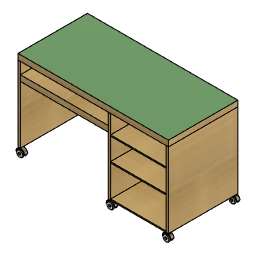
Ejercicio03jaalobuela (Autodesk Fusion 360 design; units mm, degrees)
Autodesk Fusion 360 part; units mm, degrees
box "BoxPrimitive1" add length 5 width 130 height 60 placed x (0, 0, -1) y (0, 1, 0) z (1, 0, 0) at (0, 20, 40) makes body 1
box "BoxPrimitive2" add length 70 width 60 height 2 placed x (0, 0, -1) y (-1, 0, 0) z (0, 1, 0) at (50, 0, 10) separate body makes body 2
move_body "Move1" bodies 2 to x (1, 0, 0) y (0, 1, 0) z (0, 0, 1) at (10, 20, 25)
copy_body "CopyPasteBodies1" bodies 2 makes body 3
move_body "Move2" bodies 3 to x (1, 0, 0) y (0, 1, 0) z (0, 0, 1) at (0, 128, 0)
copy_body "CopyPasteBodies2" bodies 3 makes body 4
move_body "Move3" bodies 4 to x (1, 0, 0) y (0, 1, 0) z (0, 0, 1) at (0, -50, 0)
box "BoxPrimitive3" add length 65 width 126 height 2 placed x (0, 0, -1) y (0, 1, 0) z (1, 0, 0) at (0, -161, 30) separate body makes body 5
move_body "Move4" bodies 4 to x (1, 0, 0) y (0, 1, 0) z (0, 0, 1) at (0, 0, -20)
extrude "Extrude1" cut 1 faces at (0, 98.6667, -31.6667) along direction (1, 0, 0) blind 0.2 on bodies 4 bodies 4
move_body "Move5" bodies 4 to x (1, 0, 0) y (0, 1, 0) z (0, 0, 1) at (0, 0, 20)
move_body "Move6" bodies 5 to x (1, 0, 0) y (0, 1, 0) z (0, 0, 1) at (0, 183, 5)
move_body "Move7" bodies 4 3 2 to x (1, 0, 0) y (0, 1, 0) z (0, 0, 1) at (0, 0, -75)
extrude "Extrude2" cut 3 faces at (40, 20.6667, -110) (40.0667, 98.6667, -110) (40, 148.6667, -110) along direction (0, 0, 1) blind 5 on bodies 2 3 4 bodies 2 3 4
move_body "Move8" bodies 2 3 4 to x (1, 0, 0) y (0, 1, 0) z (0, 0, 1) at (0, 0, 75)
box "BoxPrimitive4" add length 50 width 58 height 2 placed x (0, 1, 0) y (-1, 0, 0) z (0, 0, 1) at (88, 190, 0) separate body makes body 6
move_body "Move9" bodies 6 to x (1, 0, 0) y (0, 1, 0) z (0, 0, 1) at (0, -91, 0)
move_body "Move10" bodies 6 to x (1, 0, 0) y (0, 1, 0) z (0, 0, 1) at (-28, -1, -32)
move_body "Move11" bodies 6 to x (1, 0, 0) y (0, 1, 0) z (0, 0, 1) at (0, 0, -9)
extrude "Extrude3" cut 1 faces at (40.6667, 98, -40.3333) along direction (0, 1, 0) blind 2 on bodies 6 bodies 6
extrude "Extrude4" cut 1 faces at (21.3333, 116, -39) along direction (0, 0, -1) blind 1 on bodies 6 bodies 6
move_body "Move12" bodies 6 to x (1, 0, 0) y (0, 1, 0) z (0, 0, 1) at (0, 0, 11)
copy_body "CopyPasteBodies3" bodies 6 makes body 7
move_body "Move13" bodies 7 to x (1, 0, 0) y (0, 1, 0) z (0, 0, 1) at (0, 0, 28)
copy_body "CopyPasteBodies4" bodies 7 makes body 8
move_body "Move14" bodies 8 to x (1, 0, 0) y (0, 1, 0) z (0, 0, 1) at (0, 0, 20)
box "BoxPrimitive5" add length 76 width 58 height 5 placed x (0, 1, 0) y (-1, 0, 0) z (0, 0, 1) at (188, 60, 0) separate body makes body 9
move_body "Move15" bodies 9 to x (1, 0, 0) y (0, 1, 0) z (0, 0, 1) at (-128, -38, 30)
move_body "Move16" bodies 9 to x (1, 0, 0) y (0, 1, 0) z (0, 0, 1) at (0, 0, -10)
cylinder "CylinderPrimitive1" add diameter 6 height 4 placed x (0, 0, -1) y (0, 1, 0) z (1, 0, 0) at (0, 20, -33) separate body makes body 10
move_body "Move17" bodies 10 to x (1, 0, 0) y (0, 1, 0) z (0, 0, 1) at (75, 0, 0)
cylinder "CylinderPrimitive2" add diameter 2 height 4.5 placed x (0, 0, -1) y (0, 1, 0) z (1, 0, 0) at (79, 28, -25) separate body makes body 11
move_body "Move18" bodies 11 to x (1, 0, 0) y (0, 1, 0) z (0, 0, 1) at (-4.5, -8, -8)
move_body "Move19" bodies 11 to x (1, 0, 0) y (0, 1, 0) z (0, 0, 1) at (0.25, 0, 0)
box "BoxPrimitive6" add length 3 width 5 height 1 placed x (0, 1, 0) y (-1, 0, 0) z (0, 0, 1) at (131, -2, 0) separate body makes body 12
cylinder "CylinderPrimitive3" add diameter 7.5 height 4 placed x (0, 0, -1) y (0, 1, 0) z (1, 0, 0) at (0, 63, -66) separate body makes body 13
hole "Hole1" at (4, 63, -66) direction (-1, 0, 0) diameter 6 end through all bodies 13
sketch "Sketch10" plane through (4, 0, 0) normal (1, 0, 0) x (0, 1, 0)
  circle A0 centre (63, -66) radius 3
  circle A1 centre (63, -66) radius 3.75
  line L0 (58, -66) -> (70.6215, -66)
  line L1 (70.6215, -66) -> (70.6215, -70.5064)
  line L2 (70.6215, -70.5064) -> (58, -70.5064)
  line L3 (58, -70.5064) -> (58, -66)
  constraint horizontal L0
  constraint vertical L1
  constraint horizontal L2
  constraint vertical L3
move_body "Move20" bodies 13 to x (1, 0, 0) y (0, 1, 0) z (0, 0, 1) at (-2, 0, 0)
extrude "Extrude5" cut sketch "Sketch10" against normal blind 8.5 contours A0 A1 L0 | A0 L0 | A1 L0 L1 L2 L3 picked at (66.2763, -67.2056) picked at (62.6347, -68.0575) bodies 13
fillet "Fillet1" radius 0.5 1 edges at (79, 18.9152, -30.203) on bodies 10
fillet "Fillet2" radius 0.5 1 edges at (75, 21.0848, -30.203) on bodies 10
fillet "Fillet3" radius 0.2 1 edges at (79.25, 19.6384, -32.0677) on bodies 11
fillet "Fillet4" radius 0.2 1 edges at (74.75, 20.3616, -32.0677) on bodies 11
move_body "Move21" bodies 13 to x (1, 0, 0) y (0, 1, 0) z (0, 0, 1) at (76.5, -43, 30)
move_body "Move22" bodies 13 to x (1, 0, 0) y (0, 1, 0) z (0, 0, 1) at (0, 0, 3)
move_body "Move23" bodies 13 to x (1, 0, 0) y (0, 1, 0) z (0, 0, 1) at (0, 0, 4)
extrude "Extrude6" cut 1 faces at (78.5, 16.94, -27.3196) along direction (-1, 0, 0) blind 1 on bodies 13 bodies 13
move_body "Move24" bodies 13 to x (1, 0, 0) y (0, 1, 0) z (0, 0, 1) at (1, 0, -4)
fillet "Fillet5" radius 0.2 4 edges at (78.5, 20, -29.25) (77, 23.75, -33) (75.5, 20, -29.25) (77, 16.25, -33) on bodies 13
move_body "Move25" bodies 12 to x (1, 0, 0) y (0, 1, 0) z (0, 0, 1) at (-50.2, 22, -33)
move_body "Move26" bodies 12 to x (1, 0, 0) y (0, 1, 0) z (0, 0, 1) at (0, 0, 3)
move_body "Move27" bodies 12 to x (1, 0, 0) y (0, 1, 0) z (0, 0, 1) at (-2, -0.5, 1.5)
extrude "Extrude7" cut 1 faces at (73.8, 21.5, -28.1667) along direction (1, 0, 0) blind 2 on bodies 12 bodies 12
extrude "Extrude8" cut 1 faces at (76.8, 20.5, -27.5) along direction (0, 0, -1) blind 0.5 on bodies 12 bodies 12
move_body "Move28" bodies 12 to x (1, 0, 0) y (0, 1, 0) z (0, 0, 1) at (0, -0.5, -0.5)
extrude "Extrude9" add 1 faces at (77.8, 19, -28.8333) along direction (0, -1, 0) blind 0.5 on bodies 12 bodies 12
move_body "Move29" bodies 12 13 10 11 to x (1, 0, 0) y (0, 1, 0) z (0, 0, 1) at (-18, 0, -3.5)
move_body "Move30" bodies 12 to x (1, 0, 0) y (0, 1, 0) z (0, 0, 1) at (0, 0, -0.25)
move_body "Move31" bodies 12 11 13 10 to x (1, 0, 0) y (0, 1, 0) z (0, 0, 1) at (-0.8, 1.5, 2.25)
copy_body "CopyPasteBodies5" bodies 13 10 11 12 makes body 14 makes body 15 makes body 16 makes body 17
move_body "Move32" bodies 14 15 16 17 to x (1, 0, 0) y (0, 1, 0) z (0, 0, 1) at (-57, 0, 0)
copy_body "CopyPasteBodies6" bodies 13 10 11 makes body 18 makes body 19 makes body 20
move_body "Move33" bodies 18 19 20 12 to x (1, 0, 0) y (0, 1, 0) z (0, 0, 1) at (0, 78, 0)
copy_body "CopyPasteBodies7" bodies 20 18 19 12 makes body 21 makes body 22 makes body 23 makes body 24
move_body "Move34" bodies 21 22 23 24 to x (1, 0, 0) y (0, 1, 0) z (0, 0, 1) at (0, 48.5, 0)
copy_body "CopyPasteBodies8" bodies 22 21 23 18 19 20 24 12 makes body 25 makes body 26 makes body 27 makes body 28 makes body 29 makes body 30 makes body 31 makes body 32
move_body "Move35" bodies 25 26 27 28 29 30 31 32 to x (1, 0, 0) y (0, 1, 0) z (0, 0, 1) at (-60, 0, 0)
move_body "Move36" bodies 25 26 27 28 29 30 31 32 to x (1, 0, 0) y (0, 1, 0) z (0, 0, 1) at (3, 0, 0)
move_body "Move37" bodies 2 4 1 24 12 15 23 9 11 8 14 6 17 16 3 7 13 20 21 10 18 19 22 32 26 31 28 5 27 25 30 29 to x (0, -1, 0) y (1, 0, 0) z (0, 0, 1) at (-70, 20, 0)
scale "Scale1" factor 10 about (78, 20.8, -36.75) bodies 20 19 22 13 16 18 27 23 9 17 10 7 11 8 12 6 21 31 1 4 3 15 26 2 24 14 5 25 32 29 28 30
